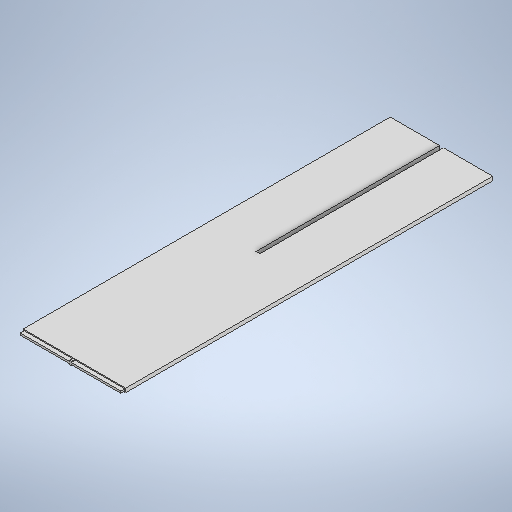
# Autodesk Inventor part: Sustainable Chair_V1 - Leg(B)_CPY
Saved by Autodesk Inventor 2025.2 (Build 292293000, 293)
## iProperties
Created: 2025-02-09
Part Number: Sustainable Chair_V1 - Leg(B)_CPY
Material: Foam Board - V3
Document SubType Name: Modeling
Designer: Dylan
Mass: 39.724 g
Surface Area: 1185.86 cm^2
Volume: 262.842 cm^3
Density: 0.151132 g/cm^3
Appearance: Default(1)
Author: VRK99-0110
Title: Sustainable Chair_V1 - Leg(B)_CPY
Subject: Sustainable Chair Project
Autodesk Inventor part; units mm, degrees
ref_plane "YZ Plane" through (0, 0, 0) normal (1, 0, 0) x (0, 1, 0)
ref_plane "XZ Plane" through (0, 0, 0) normal (0, 1, 0) x (-1, 0, 0)
ref_plane "XY Plane" through (0, 0, 0) normal (0, 0, 1) x (1, 0, 0)
sketch "Sketch1" plane through (0, 0, 0) normal (0, 1, 0) x (-1, 0, 0)
  line L0 (0, 0) -> (50, 0)
  line L1 (50, 0) -> (50, -447.675)
  line L2 (50, -447.675) -> (0, -447.675)
  line L3 (0, -447.675) -> (0, 0)
  dimension "d0" = 50
  dimension "d1" = 447.675
  constraints: 8 end point, 2 parallel, 1 horizontal, 1 perpendicular
  measures "d0" distance of L1.end L2.end
  measures "d1" distance of L0.end L1.end
extrude "Extrusion1" add sketch "Sketch1" along normal blind 4.7625
sketch "Sketch2" plane through (-50, 0, 0) normal (0, 0, 1) x (1, 0, 0)
  line L0 (1.1907, 3.5648) -> (1.1907, 1.1907)
  line L1 (50, 0) -> (0, 0) projected
  line L2 (50, 4.7625) -> (0, 4.7625) projected
  line L3 (1.1907, 1.1907) -> (48.8093, 1.1907)
  line L4 (1.1907, 3.5648) -> (48.8093, 3.5648)
  line L5 (48.8093, 3.5648) -> (48.8093, 1.1907)
  line L6 (50, 0) -> (50, 4.7625) projected
  constraints: 8 end point, 1 parallel
extrude "Extrusion2" add sketch "Sketch2" along normal blind 4.7625
sketch "Sketch3" plane through (0, 4.7625, 0) normal (0, 1, 0) x (1, 0, 0)
  line L0 (0, 0) -> (-25, 0)
  line L1 (-1.1907, 0) -> (-48.8093, 0) projected
  line L2 (-25, 65) -> (-19, 65)
  line L3 (-19, 65) -> (-25, 65)
  line L4 (-25, 65) -> (-31, 65)
  line L5 (-31, 65) -> (-31, 447.675)
  line L6 (0, 447.675) -> (-50, 447.675) projected
  line L7 (-19, 65) -> (-19, 447.675)
  line L8 (-19, 447.675) -> (-31, 447.675)
  dimension "d11" = 25
  dimension "d13" = 6
  dimension "d14" = 6
  constraints: 14 end point, 2 vertical, 1 collinear, 1 horizontal, 1 midpoint, 1 perpendicular, 1 point on line
  measures "d11" distance of L0.start L0.end
  measures "d13" distance of L2.start L2.end
  measures "d14" distance of L2.start L4.end
extrude "Extrusion3" cut sketch "Sketch3" against normal blind 10
sketch "Sketch4" plane through (-19, 4.7625, -65) normal (0, 0, -1) x (-1, 0, 0)
  line L0 (12, -4.7625) -> (0, -4.7625) projected
  line L1 (12, 0) -> (12, -4.7625) projected
  line L2 (0, 0) -> (12, 0) projected
  line L3 (0, 0) -> (0, -4.7625) projected
  point P0 (-19, -4.7625)
extrude "Extrusion4" add sketch "Sketch4" along normal blind 158.838
sketch "Sketch7" plane through (-19, 4.7625, -223.838) normal (0, 0, -1) x (-1, 0, 0)
  line L0 (0, -4.7625) -> (0, 0) projected
  line L1 (3.6185, 0) -> (3.6185, -4.7625)
  line L2 (3.6185, -4.7625) -> (8.3815, -4.7625)
  line L3 (8.3815, -4.7625) -> (8.3815, 0)
  line L4 (3.6185, 0) -> (8.3815, 0)
  line L5 (12, 0) -> (0, 0) projected
  line L6 (0, 0) -> (3.6185, 0)
  line L7 (0, -4.7625) -> (12, -4.7625) projected
  line L8 (3.6185, -4.7625) -> (0, -4.7625)
  line L9 (0, -4.7625) -> (0, 0)
  line L10 (8.3815, 0) -> (12, 0)
  line L11 (12, 0) -> (12, -4.7625) projected
  line L12 (12, 0) -> (12, -4.7625)
  line L13 (12, -4.7625) -> (8.3815, -4.7625)
  point P0 (-19, -4.7625)
  dimension "d20" = 4.763
  constraints: 20 end point, 7 collinear, 2 perpendicular
  measures "d20" distance of L1.end L2.end
extrude "Extrusion5" add sketch "Sketch7" along normal blind 223.837 contours L0 L5 L1 L7 | L3 L5 L11 L7
sketch "Sketch8" plane through (-50, 0, 0) normal (0, 0, 1) x (1, 0, 0)
  line L0 (26.187, 0) -> (26.187, 1.1907)
  line L1 (26.187, 1.1907) -> (23.813, 1.1907)
  line L2 (23.813, 1.1907) -> (23.813, 0)
  line L3 (26.187, 0) -> (23.813, 0)
  line L4 (23.813, 1.1907) -> (26.187, 1.1907)
  line L5 (1.1907, 1.1907) -> (1.1907, 3.5648) projected
  line L6 (1.1907, 2.3778) -> (48.8093, 2.3778)
  line L7 (48.8093, 1.1907) -> (1.1907, 1.1907) projected
  line L8 (26.187, 4.7555) -> (26.187, 3.5648)
  line L9 (26.187, 3.5648) -> (23.813, 3.5648)
  line L10 (23.813, 3.5648) -> (23.813, 4.7555)
  line L11 (26.187, 4.7555) -> (23.813, 4.7555)
  point P0 (0, 0)
  dimension "d25" = 2.374
  constraints: 20 end point, 4 symmetric about line, 1 midpoint, 1 parallel, 1 perpendicular
  measures "d25" distance of L0.end L1.end
extrude "Extrusion6" add sketch "Sketch8" along normal up to surface (4.7625 mm away)
sketch "Sketch9" plane through (0, 4.7625, 0) normal (0, 1, 0) x (1, 0, 0)
  line L0 (0, 0) -> (25, 0)
  line L1 (0, 447.675) -> (-22.6185, 447.675) projected
  line L2 (0, 447.675) -> (25, 447.675)
  line L3 (25, 447.675) -> (25, 0)
  line L4 (0, 0) -> (0, 447.675) projected
  line L5 (0, 0) -> (0, 447.675)
  line L6 (-50, 0) -> (0, 0) projected
  line L7 (-50, 0) -> (-75, 0)
  line L8 (-50, 447.675) -> (-75, 447.675)
  line L9 (-75, 447.675) -> (-75, 0)
  line L10 (-50, 0) -> (-50, 447.675)
  dimension "d28" = 25
  constraints: 16 end point, 2 horizontal, 1 collinear, 1 perpendicular
  measures "d28" distance of L0.start L0.end
extrude "Extrusion7" add sketch "Sketch9" against normal up to surface (4.7625 mm away)
sketch "Sketch10" plane through (0, 4.7625, 0) normal (0, 1, 0) x (1, 0, 0)
  line L0 (25, 0) -> (25, 447.675) projected
  line L1 (25, 0) -> (37.5, 0)
  line L2 (25, 447.675) -> (37.5, 447.675)
  line L3 (37.5, 447.675) -> (37.5, 0)
  line L4 (-75, 0) -> (25, 0) projected
  line L5 (25, 447.675) -> (-22.6185, 447.675) projected
  line L6 (25, 447.675) -> (25, 0)
  line L7 (-75, 0) -> (-75, 447.675)
  line L8 (-75, 0) -> (-87.5, 0)
  line L9 (-75, 447.675) -> (-87.5, 447.675)
  line L10 (-87.5, 447.675) -> (-87.5, 0)
  point P0 (0, 0)
  dimension "d31" = 12.5
  constraints: 16 end point, 2 horizontal, 1 collinear, 1 perpendicular
  measures "d31" distance of L0.start L1.end
extrude "Extrusion8" add sketch "Sketch10" against normal up to surface (4.7625 mm away)
sketch "Sketch11" plane through (-48.8093, 1.1907, 0) normal (0, 0, 1) x (1, 0, 0)
  line L0 (47.6185, 0) -> (24.9963, 0) projected
  line L1 (47.6185, 0) -> (85.1183, 0)
  line L2 (24.9963, 2.374) -> (47.6185, 2.374) projected
  line L3 (47.6185, 2.374) -> (85.1183, 2.374)
  line L4 (85.1183, 2.374) -> (85.1183, 0)
  line L5 (24.9963, -1.1907) -> (22.6223, -1.1907) projected
  line L6 (23.8093, -1.1907) -> (23.8093, 3.5648)
  line L7 (22.6223, 3.5648) -> (24.9963, 3.5648) projected
  line L8 (47.6185, 2.374) -> (47.6185, 0) projected
  line L9 (47.6185, 2.374) -> (47.6185, 0)
  line L10 (0, 0) -> (-37.4998, 0)
  line L11 (0, 2.374) -> (-37.4998, 2.374)
  line L12 (-37.4998, 2.374) -> (-37.4998, 0)
  line L13 (0, 2.374) -> (0, 0)
  point P0 (48.8093, -1.1907)
  constraints: 18 end point, 4 symmetric about line, 2 midpoint, 1 collinear, 1 horizontal, 1 perpendicular
extrude "Extrusion9" add sketch "Sketch11" along normal up to surface (4.7625 mm away)
body "Solid1"
